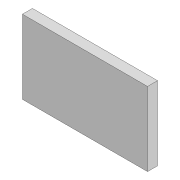
# Autodesk Inventor part: Display_B
Saved by Autodesk Inventor 2020 (Build 240168000, 168)
## iProperties
Created: 2021-11-28
Part Number: Display_B
Material: 一般
Document SubType Name: Modeling
Designer: ken113
Density: 1 g/cm^3
Appearance: 既定
Author: ken113
Autodesk Inventor part; units mm, degrees
ref_plane "YZ Plane" through (0, 0, 0) normal (1, 0, 0) x (0, 1, 0)
ref_plane "XZ Plane" through (0, 0, 0) normal (0, 1, 0) x (-1, 0, 0)
ref_plane "XY Plane" through (0, 0, 0) normal (0, 0, 1) x (1, 0, 0)
sketch "スケッチ1" plane through (0, 0, 0) normal (0, 0, 1) x (1, 0, 0)
  line L0 (369, -217.5) -> (-369, -217.5)
  line L1 (-369, -217.5) -> (-369, 217.5)
  line L2 (-369, 217.5) -> (369, 217.5)
  line L3 (369, 217.5) -> (369, -217.5)
  line L4 (369, -217.5) -> (-369, 217.5) construction
  line L5 (-369, -217.5) -> (369, 217.5) construction
  point P0 (0, 0)
  dimension "d0" = 738
  dimension "d1" = 435
  constraints: 12 end point, 2 midpoint, 2 parallel, 1 horizontal, 1 perpendicular
  measures "d0" distance of L1.end L2.end
  measures "d1" distance of L0.end L1.end
extrude "押し出し1" add sketch "スケッチ1" along normal blind 59
